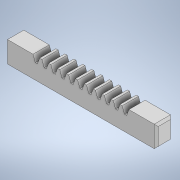
# Autodesk Inventor part: Ch7(5) Part 11 Rack
Saved by Autodesk Inventor 2020 (Build 240168000, 168)
## iProperties
Created: 2021-03-04
Part Number: Ch7(5) Part 11 Rack
Material: Generic
Document SubType Name: Modeling
Designer: adriggs
Density: 1 g/cm^3
Appearance: Default
Author: adriggs
Autodesk Inventor part; units mm, degrees
ref_plane "YZ Plane" through (0, 0, 0) normal (1, 0, 0) x (0, 1, 0)
ref_plane "XZ Plane" through (0, 0, 0) normal (0, 1, 0) x (-1, 0, 0)
ref_plane "XY Plane" through (0, 0, 0) normal (0, 0, 1) x (1, 0, 0)
sketch "Sketch1" plane through (0, 0, 0) normal (0, 0, 1) x (1, 0, 0)
  line L0 (-77.7875, 0) -> (77.7875, 0) projected
  line L1 (0, -3.175) -> (0, 19.05) projected
  line L2 (-55.5625, 0) -> (55.5625, 0)
  line L3 (-55.5625, 0) -> (-55.5625, 15.875)
  line L4 (-55.5625, 15.875) -> (55.5625, 15.875)
  line L5 (55.5625, 15.875) -> (55.5625, 0)
  point P0 (0, 0)
  point P1 (0, 0)
  dimension "d0" = 111.125
  dimension "d1" = 15.875
  constraints: 8 end point, 3 perpendicular, 2 coincident, 1 midpoint, 1 vertical
  measures "d0" distance of L2.start L2.end
  measures "d1" distance of L2.start L3.end
extrude "Extrusion1" add sketch "Sketch1" against normal blind 12.1285
sketch "Sketch2" plane through (0, 0, 0) normal (0, 0, 1) x (1, 0, 0)
  line L0 (-55.5625, 15.875) -> (55.5625, 15.875) projected
  line L1 (-55.5625, 15.875) -> (-36.5125, 15.875)
  line L2 (-36.5125, 15.875) -> (-34.8577, 11.3284)
  line L3 (-34.8577, 11.3284) -> (-33.1851, 11.3284)
  line L4 (-33.1851, 11.3284) -> (-31.5303, 15.875)
  line L5 (-31.5303, 15.875) -> (-29.8577, 15.875)
  line L6 (55.5625, 15.875) -> (-55.5625, 15.875) construction
  line L7 (-55.5625, 15.875) -> (-55.5625, 0) projected
  line L8 (55.5625, 15.875) -> (36.5125, 15.875)
  line L9 (-29.845, 15.875) -> (-28.1902, 11.3284)
  line L10 (-28.1902, 11.3284) -> (-26.5176, 11.3284)
  line L11 (-26.5176, 11.3284) -> (-24.8628, 15.875)
  line L12 (-24.8628, 15.875) -> (-23.1902, 15.875)
  line L13 (-23.1775, 15.875) -> (-21.5227, 11.3284)
  line L14 (-21.5227, 11.3284) -> (-19.8501, 11.3284)
  line L15 (-19.8501, 11.3284) -> (-18.1953, 15.875)
  line L16 (-18.1953, 15.875) -> (-16.5227, 15.875)
  line L17 (-16.51, 15.875) -> (-14.8552, 11.3284)
  line L18 (-14.8552, 11.3284) -> (-13.1826, 11.3284)
  line L19 (-13.1826, 11.3284) -> (-11.5278, 15.875)
  line L20 (-11.5278, 15.875) -> (-9.8552, 15.875)
  line L21 (-9.8425, 15.875) -> (-8.1877, 11.3284)
  line L22 (-8.1877, 11.3284) -> (-6.5151, 11.3284)
  line L23 (-6.5151, 11.3284) -> (-4.8603, 15.875)
  line L24 (-4.8603, 15.875) -> (-3.1877, 15.875)
  line L25 (-3.175, 15.875) -> (-1.5202, 11.3284)
  line L26 (-1.5202, 11.3284) -> (0.1524, 11.3284)
  line L27 (0.1524, 11.3284) -> (1.8072, 15.875)
  line L28 (1.8072, 15.875) -> (3.4798, 15.875)
  line L29 (3.4925, 15.875) -> (5.1473, 11.3284)
  line L30 (5.1473, 11.3284) -> (6.8199, 11.3284)
  line L31 (6.8199, 11.3284) -> (8.4747, 15.875)
  line L32 (8.4747, 15.875) -> (10.1473, 15.875)
  line L33 (10.16, 15.875) -> (11.8148, 11.3284)
  line L34 (11.8148, 11.3284) -> (13.4874, 11.3284)
  line L35 (13.4874, 11.3284) -> (15.1422, 15.875)
  line L36 (15.1422, 15.875) -> (16.8148, 15.875)
  line L37 (16.8275, 15.875) -> (18.4823, 11.3284)
  line L38 (18.4823, 11.3284) -> (20.1549, 11.3284)
  line L39 (20.1549, 11.3284) -> (21.8097, 15.875)
  line L40 (21.8097, 15.875) -> (23.4823, 15.875)
  line L41 (23.495, 15.875) -> (25.1498, 11.3284)
  line L42 (25.1498, 11.3284) -> (26.8224, 11.3284)
  line L43 (26.8224, 11.3284) -> (28.4772, 15.875)
  line L44 (28.4772, 15.875) -> (30.1498, 15.875)
  line L45 (30.1625, 15.875) -> (31.8173, 11.3284)
  line L46 (31.8173, 11.3284) -> (33.4899, 11.3284)
  line L47 (33.4899, 11.3284) -> (35.1447, 15.875)
  line L48 (35.1447, 15.875) -> (36.8173, 15.875)
  point P0 (0, 0)
  point P1 (-35.6851, 13.6017)
  point P2 (-32.3577, 13.6017)
  point P3 (-29.0176, 13.6017)
  point P4 (-25.6902, 13.6017)
  point P5 (-22.3501, 13.6017)
  point P6 (-19.0227, 13.6017)
  point P7 (-15.6826, 13.6017)
  point P8 (-12.3552, 13.6017)
  point P9 (-9.0151, 13.6017)
  point P10 (-5.6877, 13.6017)
  point P11 (-2.3476, 13.6017)
  point P12 (0.9798, 13.6017)
  point P13 (4.3199, 13.6017)
  point P14 (7.6473, 13.6017)
  point P15 (10.9874, 13.6017)
  point P16 (14.3148, 13.6017)
  point P17 (17.6549, 13.6017)
  point P18 (20.9823, 13.6017)
  point P19 (24.3224, 13.6017)
  point P20 (27.6498, 13.6017)
  point P21 (30.9899, 13.6017)
  point P22 (34.3173, 13.6017)
  dimension "d4" = 19.05
  dimension "d5" = 6.6548
  dimension "d6" = 20
  dimension "d7" = 4.5466
  dimension "d12" = 6.6675
  constraints: 92 end point, 71 horizontal alignment, 21 parallel, 20 collinear, 3 point on line, 2 equal length, 2 midpoint, 2 other
  measures "d4" distance of L1.start L1.end
  measures "d5" distance of L5.end L1.end
  measures "d6" angle of L2 L7
  measures "d12" distance of L1.end L9.start
extrude "Extrusion2" cut sketch "Sketch2" against normal through all
sketch "Sketch3" plane through (-55.5625, 0, 0) normal (-1, 0, 0) x (0, 0, 1)
  circle A0 centre (-6.0642, 7.9375) radius 3.175
  line L0 (-12.1285, 0) -> (-12.1285, 15.875) projected
  line L1 (0, 15.875) -> (-12.1285, 15.875) projected
  point P0 (0, 0)
  point P1 (-12.1285, 7.9375)
  point P2 (-6.0642, 15.875)
  dimension "d19" = 6.35
  constraints: 2 midpoint, 1 centre point, 1 horizontal alignment, 1 vertical alignment
  measures "d19" diameter of A0
extrude "Extrusion3" cut sketch "Sketch3" against normal blind 15.875
chamfer "Chamfer1" distance 1.524 angle 45 4 edges at (55.5625, 15.875, -6.0642) (55.5625, 7.9375, 0) (55.5625, 0, -6.0642) (55.5625, 7.9375, -12.1285)
body "Solid1"
